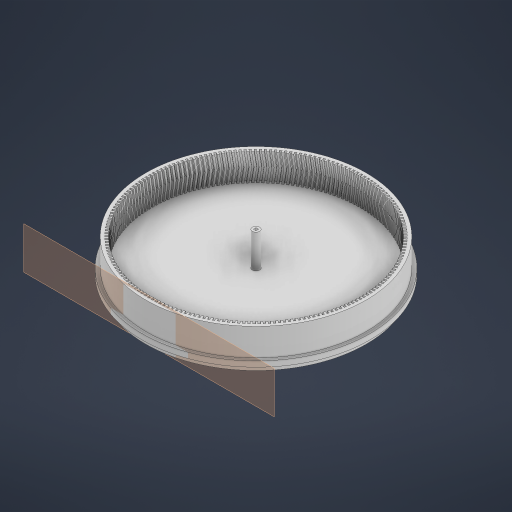
# Autodesk Inventor part: electronics-cover
Saved by Autodesk Inventor 2023 (Build 270158030, 158C)
## iProperties
Created: 2022-05-14
Part Number: electronics-cover
Material: Generic
Document SubType Name: Modeling
Designer: jayso
Density: 1 g/cm^3
Appearance: Default
Author: jayso
Autodesk Inventor part; units mm, degrees
ref_plane "YZ Plane" through (0, 0, 0) normal (1, 0, 0) x (0, 1, 0)
ref_plane "XZ Plane" through (0, 0, 0) normal (0, 1, 0) x (-1, 0, 0)
sketch "Sketch2" plane through (0, 0, 0) normal (0, 1, 0) x (-1, 0, 0)
  circle A0 centre (0, 0) radius 125
  dimension "d0" = 250
  constraints: 1 centre point, 1 coincident
  measures "d0" diameter of A0
extrude "Extrusion1" add sketch "Sketch2" along normal blind 6
sketch "Sketch3" plane through (0, 0, 0) normal (0, -1, 0) x (1, 0, 0)
  circle A0 centre (0, 0) radius 121
  dimension "d3" = 242
  constraints: 1 centre point, 1 coincident
  measures "d3" diameter of A0
extrude "Extrusion2" add sketch "Sketch3" along normal blind 6
sketch "Sketch4" plane through (0, 6, 0) normal (0, 1, 0) x (1, 0, 0)
  circle A0 centre (0, 0) radius 4
  dimension "d6" = 8
  constraints: 1 centre point, 1 coincident
  measures "d6" diameter of A0
extrude "Extrusion3" add sketch "Sketch4" along normal blind 8
sketch "Sketch6" plane through (0, 14, 0) normal (0, 1, 0) x (1, 0, 0)
  line L0 (-1.5, 1.5) -> (1.5, 1.5)
  line L1 (1.5, 1.5) -> (1.5, -1.5)
  line L2 (1.5, -1.5) -> (-1.5, -1.5)
  line L3 (-1.5, -1.5) -> (-1.5, 1.5)
  circle A0 centre (0, 0) radius 4 projected
  point P0 (-1.5, 0)
  point P1 (0, 1.5)
  dimension "d9" = 3
  dimension "d10" = 3
  dimension "d11" = 1.5
  dimension "d12" = 1.5
  constraints: 8 end point, 2 midpoint, 2 parallel, 1 horizontal, 1 perpendicular
  measures "d9" distance of L0.end L1.end
  measures "d10" distance of L1.end L2.end
  measures "d11" distance of A0.centre point (-1.5, 0)
  measures "d12" distance of A0.centre point (0, 1.5)
extrude "Extrusion4" cut sketch "Sketch6" against normal blind 34.9875 contours L0 L1 L2 L3
sketch "Sketch9" plane through (0, 6, 0) normal (0, 1, 0) x (1, 0, 0)
  circle A0 centre (0, 0) radius 121
  constraints: 1 centre point, 1 coincident
extrude "Extrusion5" add sketch "Sketch9" along normal blind 30
sketch "Sketch12" plane through (0, 36, 0) normal (0, 1, 0) x (1, 0, 0)
  circle A0 centre (0, 0) radius 117.5
  dimension "d17" = 235
  constraints: 1 centre point, 1 coincident
  measures "d17" diameter of A0
extrude "Extrusion6" cut sketch "Sketch12" against normal blind 30
ref_plane "Work Plane2" through (0, 0, 117.5) normal (0, 0, 1) x (1, 0, 0)
sketch "Sketch17" plane through (0, 0, 117.5) normal (0, 0, 1) x (1, 0, 0)
  line L0 (-117.5, 36) -> (117.5, 36) projected
  line L1 (0, 36) -> (0, 6)
  line L2 (-117.5, 6) -> (117.5, 6) projected
  line L3 (0, 21) -> (-2, 21)
  line L4 (-2, 21) -> (0, 6)
  line L5 (0, 36) -> (-2, 21)
  line L6 (0, 6) -> (2, 6)
  line L7 (0, 36) -> (2, 36)
  line L8 (2, 36) -> (0, 21)
  line L9 (2, 6) -> (0, 21)
  point P0 (0, 0)
  dimension "d25" = 2
  dimension "d26" = 2
  dimension "d27" = 2
  constraints: 16 end point, 3 midpoint, 2 point on line, 1 horizontal
  measures "d25" distance of L3.start L3.end
  measures "d26" distance of L1.end L6.end
  measures "d27" distance of L1.start L7.end
extrude "Extrusion8" add sketch "Sketch17" against normal blind 3
pattern_circular "Circular Pattern1" count 185 over 360 about axis through (0, 36, 0) along (0, -1, 0) of "Extrusion8"
sketch "Sketch22" plane through (0, 6, 0) normal (0, 1, 0) x (1, 0, 0)
  circle A0 centre (0, 0) radius 4
  dimension "d33" = 8
  constraints: 1 centre point, 1 coincident
  measures "d33" diameter of A0
extrude "Extrusion9" add sketch "Sketch22" along normal blind 36.9
sketch "Sketch23" plane through (0, 42.9, 0) normal (0, 1, 0) x (1, 0, 0)
  line L0 (-1.5, 1.5) -> (-1.5, -1.5) projected
  line L1 (1.5, -1.5) -> (1.5, 1.5) projected
  line L2 (-1.5, 1.5) -> (1.5, 1.5)
  line L3 (1.5, 1.5) -> (1.5, -1.5)
  line L4 (1.5, -1.5) -> (-1.5, -1.5)
  line L5 (-1.5, -1.5) -> (-1.5, 1.5)
  point P0 (0, 0)
  constraints: 8 end point, 2 parallel, 1 horizontal, 1 perpendicular
extrude "Extrusion10" cut sketch "Sketch23" against normal blind 134.775
body "Solid1"
